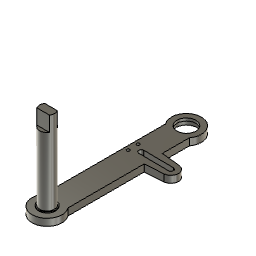
primary-arm (Autodesk Fusion 360 design; units mm, degrees)
Autodesk Fusion 360 part; units mm, degrees
note: some values were not read from the file. Chosen so that the rebuilt part matches the saved one: which face or edge a step refers to; a direction. Set by a fixed rule: which sketch regions a step uses.
sketch "Sketch1" plane through (0, 0, 0) normal (0, 0, 1) x (1, 0, 0)
  line L0 (0, 0) -> (0, 139.5) construction
  line L1 (-12, 130.5) -> (-12, 9)
  line L2 (12, 9) -> (12, 130.5)
  line L3 (-12, 69.75) -> (12, 69.75) construction
  circle A0 centre (0, 139.5) radius 10.7
  arc A1 (12, 130.5) -> (-12, 130.5) centre (0, 139.5) ccw
  arc A2 (-12, 9) -> (12, 9) centre (0, 0) ccw
  point P0 (0, 69.75)
  dimension "d1" = 139.5
  dimension "d2" = 30
  dimension "d3" = 24
  dimension "d4" = 21.4
  constraint coincident L0.start A2.centre
  constraint equal A1 A2
  constraint coincident L0.end A0.centre
  constraint vertical L0
  constraint vertical L1
  constraint parallel L0 L2
  constraint midpoint L1 L3.start
  constraint midpoint L2 L3.end
  constraint midpoint L0 P0
  constraint midpoint L3 P0
  constraint concentric A0 A1
  measures "d1" distance of L0.start L0.end
  measures "d2" diameter of A2
  measures "d3" distance of L1 L2
  measures "d4" diameter of A0
extrude "Extrude1" add sketch "Sketch1" along normal blind 7
ref_plane "WorkPlane1" through (0, 0, 4.3) normal (0, 0, 1) x (1, 0, 0)
sketch "Sketch2" plane through (0, 0, 4.3) normal (0, 0, 1) x (1, 0, 0)
  circle A0 centre (0, 139.5) radius 9.5
  circle A1 centre (0, 139.5) radius 10.7
  dimension "d8" = 19
  constraint concentric A0 A1
  measures "d8" diameter of A0
extrude "Extrude2" add sketch "Sketch2" along normal up to surface (2.7 mm away)
sketch "Sketch3" plane through (0, 0, 7) normal (0, 0, 1) x (-1, 0, 0)
  circle A0 centre (0, -139.5) radius 9.5
  arc A1 (12, -9) -> (-12, -9) centre (0, 0) ccw
  line L0 (-12, -9) -> (-12, -130.5)
  arc A2 (-12, -130.5) -> (12, -130.5) centre (0, -139.5) ccw
  line L1 (12, -130.5) -> (12, -9)
  circle A3 centre (0, 0) radius 8.5
  dimension "d11" = 17
  constraint coincident A1.centre A3.centre
  measures "d11" diameter of A3
extrude "Extrude3" add sketch "Sketch3" along normal blind 1 contours A3
sketch "Sketch4" plane through (0, 0, 8) normal (0, 0, 1) x (-1, 0, 0)
  circle A0 centre (0, 0) radius 8.5
  circle A1 centre (0, 0) radius 7.45
  dimension "d14" = 14.9
  constraint coincident A0.centre A1.centre
  measures "d14" diameter of A1
extrude "Extrude4" add sketch "Sketch4" along normal blind 68 contours A1
sketch "Sketch5" plane through (0, 0, 76) normal (0, 0, 1) x (-1, 0, 0)
  circle A0 centre (0, 0) radius 7.45
  line L0 (0, 3.9) -> (0, -3.9) construction
  line L1 (6.3476, -3.9) -> (-6.3476, -3.9)
  line L2 (6.3476, 3.9) -> (-6.3476, 3.9)
  arc A1 (6.3476, -3.9) -> (6.3476, 3.9) centre (0, 0) ccw
  arc A2 (-6.3476, 3.9) -> (-6.3476, -3.9) centre (0, 0) ccw
  dimension "d18" = 7.8
  constraint coincident A0.centre A1.centre
  constraint equal A0 A1
  constraint vertical L0
  constraint midpoint A0.centre L0
  constraint coincident A0 L1.start
  constraint coincident A0 L1.end
  constraint horizontal L1
  constraint coincident L2.end A1
  constraint perpendicular L0 L2
  constraint coincident L0.end L1
  constraint coincident L0.start L2
  constraint concentric A1 A2
  measures "d18" distance of L0.start L0.end
extrude "Extrude5" add sketch "Sketch5" along normal blind 15 contours A0 L1 L2 A1 A2
sketch "Sketch6" plane through (0, 0, 7) normal (0, 0, 1) x (-1, 0, 0)
  circle A0 centre (0, 0) radius 8.5
  circle A1 centre (0, -139.5) radius 9.5
  arc A2 (12, -9) -> (-12, -9) centre (0, 0) ccw
  line L0 (-12, -9) -> (-12, -130.5)
  arc A3 (-12, -130.5) -> (12, -130.5) centre (0, -139.5) ccw
  line L1 (12, -130.5) -> (12, -9)
  line L2 (12, -104.5) -> (7, -104.5)
  line L3 (7, -104.5) -> (7, -84.5)
  line L4 (7, -84.5) -> (12, -84.5)
  line L5 (12, -84.5) -> (12, -104.5)
  dimension "d21" = 20
  dimension "d22" = 5
  dimension "d23" = 35
  constraint horizontal L2
  constraint vertical L3
  constraint horizontal L4
  constraint vertical L5
  constraint coincident L1 L2.start
  measures "d21" distance of L2.start L4.end
  measures "d22" distance of L2.start L2.end
  measures "d23" vertical distance of A1.centre L2.end
sketch "Sketch7" plane through (0, 0, 0) normal (0, 0, 1) x (1, 0, 0)
  circle A0 centre (30, 94) radius 2.55
  line L0 (0, 94) -> (30, 94) construction
  line L1 (0.0017, 104.5) -> (30.7373, 101.4637)
  line L2 (0.0017, 84.5) -> (30.4949, 86.5163)
  arc A1 (30.4949, 86.5163) -> (30.7373, 101.4637) centre (30, 94) ccw
  line L3 (0.0017, 104.5) -> (0.0017, 84.5)
  line L4 (0.0017, 104.5) -> (-12.0003, 104.5)
  line L5 (-12.0003, 104.5) -> (-12.0003, 84.2074)
  line L6 (-12.0003, 84.2074) -> (0.0017, 84.5)
  line L7 (0.0017, 91.5) -> (0.0017, 96.5)
  line L8 (30.0047, 91.45) -> (30.0047, 96.55)
  point P0 (0.0017, 104.5)
  point P1 (0, 139.5)
  point P2 (-8, 94)
  dimension "d24" = 35
  dimension "d25" = 20
  dimension "d26" = 5.1
  dimension "d27" = 30
  dimension "d28" = 15
  constraint concentric A0 A1
  constraint coincident A0.centre L0.end
  constraint coincident P0 L1.start
  constraint tangent L1 A1
  constraint tangent L2 A1
  constraint perpendicular L3 L4
  constraint perpendicular L4 L5
  constraint coincident L3 L7.start
  constraint coincident L3 L7.end
  constraint coincident A0 L8.start
  constraint coincident A0 L8.end
  constraint perpendicular L0 L8
  constraint horizontal L0.start P2
  constraint horizontal L0
  constraint vertical L3
  measures "d24" distance of P0 P1
  measures "d25" distance of P0 L2.start
  measures "d26" diameter of A0
  measures "d27" distance of L0.start A0.centre
  measures "d28" diameter of A1
extrude "Extrude6" add sketch "Sketch7" along normal blind 7 contours L1 L2 A1 L3 L7
sketch "Sketch10" plane through (0, 0, 7) normal (0, 0, 1) x (-1, 0, 0)
  circle A0 centre (-30, -94) radius 2.55
  line L0 (-12, -103.3147) -> (-12, -130.5)
  arc A1 (-12, -130.5) -> (12, -130.5) centre (0, -139.5) ccw
  arc A2 (12, -9) -> (-12, -9) centre (0, 0) ccw
  line L1 (-12, -9) -> (-12, -85.2934)
  line L2 (-12, -85.2934) -> (-30.4949, -86.5163)
  arc A3 (-30.4949, -86.5163) -> (-30.7373, -101.4637) centre (-30, -94) ccw
  line L3 (-30.7373, -101.4637) -> (-12, -103.3147)
  circle A4 centre (0, 0) radius 8.5
  circle A5 centre (0, -139.5) radius 9.5
  line L4 (-12, -103.3147) -> (-12, -85.2934) construction
  line L5 (-12, -94.304) -> (12, -94.304) construction
  line L6 (12, -130.5) -> (12, -9) construction
  circle A6 centre (8, -99.304) radius 1.5
  circle A7 centre (8, -89.304) radius 1.5
  line L7 (8, -99.304) -> (8, -89.304) construction
  line L8 (-30.0258, -96.5499) -> (-0.0274, -96.8539)
  arc A8 (-0.0274, -96.8539) -> (0.0243, -91.7542) centre (-0.0015, -94.304) ccw
  line L9 (0.0243, -91.7542) -> (-29.9742, -91.4501)
  arc A9 (-29.9742, -91.4501) -> (-30.0258, -96.5499) centre (-30, -94) ccw
  line L10 (-30, -94) -> (-0.0015, -94.304) construction
  line L11 (7, -89) -> (7, -99) construction
  point P0 (8, -94.304)
  point P1 (7, -94)
  dimension "d49" = 3
  dimension "d50" = 4
  dimension "d51" = 10
  dimension "d52" = 5
  dimension "d54" = 30
  constraint coincident L0.start L3.end
  constraint coincident L1.end L2.start
  constraint midpoint L4 L5.start
  constraint horizontal L5
  constraint coincident L5.end L6
  constraint equal A6 A7
  constraint coincident A6.centre L7.start
  constraint coincident A7.centre L7.end
  constraint vertical L7
  constraint midpoint L7 P0
  constraint coincident L5 P0
  constraint tangent L8 A8
  constraint tangent A8 L9
  constraint parallel L8 L9
  constraint tangent L9 A9
  constraint tangent L8 A9
  constraint coincident L5 A8.centre
  constraint coincident A0.centre A3.centre
  constraint equal A0 A9
  constraint vertical L11
  constraint midpoint L11 P1
  measures "d49" diameter of A6
  measures "d50" distance of L5.end L7
  measures "d51" distance of A6.centre A7.centre
  measures "d52" distance of L5.end L11
  measures "d54" distance of A0.centre A8.centre
extrude "Extrude11" cut sketch "Sketch10" against normal through all contours A0 L8 A8 L9 | A6 | A7
extrude "Extrude10" [suppressed]
extrude "Extrude7" [suppressed]
extrude "Extrude8" [suppressed]
sketch "Sketch9" plane through (0, 0, 26) normal (0, 0, 1) x (-1, 0, 0)
  circle A0 centre (-35, -94) radius 2.5
  line L0 (0, -84) -> (-35.5304, -86.5188)
  arc A1 (-35.5304, -86.5188) -> (-35.5304, -101.4812) centre (-35, -94) ccw
  line L1 (-35.5304, -101.4812) -> (0, -104)
  line L2 (0, -104) -> (12, -104)
  line L3 (12, -104) -> (12, -84)
  line L4 (12, -84) -> (0, -84)
  line L5 (-35, -94) -> (0, -94) construction
  line L6 (0, -84) -> (0, -104) construction
  line L7 (0, -96.5) -> (-35, -96.5)
  line L8 (-35, -91.5) -> (0, -91.5)
  arc A2 (0, -96.5) -> (0, -91.5) centre (0, -94) ccw
  arc A3 (-35, -91.5) -> (-35, -96.5) centre (-35, -94) ccw
  dimension "d42" = 5
  constraint concentric A0 A3
  constraint coincident A0.centre A1.centre
  constraint horizontal L5
  constraint coincident L5.end A2.centre
  constraint coincident L0.start L4.end
  constraint coincident L1.end L2.start
  constraint coincident L6 L7.start
  constraint coincident A0 L7.end
  constraint tangent A0 L7
  constraint perpendicular L6 L7
  constraint coincident L6 L8.end
  constraint tangent L8 A2
  measures "d42" diameter of A2
extrude "Extrude9" [suppressed]
